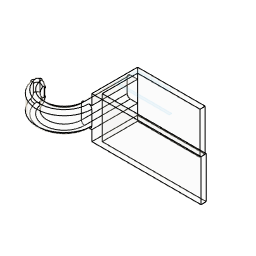
DeskHook v3 (Autodesk Fusion 360 design; units mm, degrees)
Autodesk Fusion 360 part; units mm, degrees
sketch "Sketch1" plane through (0, 0, 0) normal (0, 0, 1) x (1, 0, 0)
  line L0 (5.7833, 3.3448) -> (5.7833, 20.3448)
  line L1 (5.7833, 20.3448) -> (35.7833, 20.3448)
  line L2 (5.7833, 3.3448) -> (55.7833, 3.3448)
  line L3 (35.7833, 20.3448) -> (5.7833, 20.3448)
  line L4 (5.7833, 20.3448) -> (5.7833, 22.8448)
  line L5 (5.7833, 22.8448) -> (35.7833, 22.8448)
  line L6 (35.7833, 22.8448) -> (35.7833, 20.3448)
  line L7 (5.7833, 3.3448) -> (55.7833, 3.3448)
  line L8 (55.7833, 3.3448) -> (55.7833, 0.8448)
  line L9 (55.7833, 0.8448) -> (5.7833, 0.8448)
  line L10 (5.7833, 0.8448) -> (5.7833, 3.3448)
  line L11 (5.7833, 22.8448) -> (3.2833, 22.8448)
  line L12 (3.2833, 22.8448) -> (3.2833, 0.8448)
  line L13 (3.2833, 0.8448) -> (5.7833, 0.8448)
  line L14 (5.7833, 0.8448) -> (5.7833, 22.8448)
  dimension "d1" = 17
  dimension "d2" = 30
  dimension "d3" = 50
  dimension "d4" = 2.5
  dimension "d5" = 2.5
  dimension "d6" = 2.5
  constraint vertical L0
  constraint perpendicular L0 L1
  constraint perpendicular L0 L2
  constraint horizontal L3
  constraint vertical L4
  constraint horizontal L5
  constraint vertical L6
  constraint horizontal L7
  constraint vertical L8
  constraint horizontal L9
  constraint vertical L10
  constraint horizontal L11
  constraint vertical L12
  constraint horizontal L13
  constraint vertical L14
  measures "d1" distance of L0.start L0.end
  measures "d2" distance of L0.end L1.end
  measures "d3" distance of L0.start L2.end
  measures "d4" distance of L1.end L5.end
  measures "d5" distance of L0.start L9.end
  measures "d6" distance of L4.end L11.end
extrude "Extrude1" add sketch "Sketch1" along normal blind 20
sketch "Sketch2" plane through (0, 0, 20) normal (0, 0, 1) x (-1, 0, 0)
  line L0 (-35.7833, -22.8448) -> (-3.2833, -22.8448)
  line L1 (-3.2833, -22.8448) -> (-3.2833, -0.8448)
  line L2 (-3.2833, -0.8448) -> (-55.7833, -0.8448)
  line L3 (-55.7833, -0.8448) -> (-55.7833, -3.3448)
  line L4 (-55.7833, -3.3448) -> (-5.7833, -3.3448)
  line L5 (-5.7833, -3.3448) -> (-5.7833, -20.3448)
  line L6 (-5.7833, -20.3448) -> (-35.7833, -20.3448)
  line L7 (-35.7833, -20.3448) -> (-35.7833, -22.8448)
sketch "Sketch3" plane through (3.2833, 0, 0) normal (-1, 0, 0) x (0, -1, 0)
  line L0 (-22.8448, 0) -> (-0.8448, 0)
  line L1 (-0.8448, 0) -> (-0.8448, 20)
  line L2 (-0.8448, 20) -> (-22.8448, 20)
  line L3 (-22.8448, 20) -> (-22.8448, 0)
  line L4 (-22.8448, 5) -> (-0.8448, 5)
  line L5 (-0.8448, 5) -> (-0.8448, 15)
  line L6 (-0.8448, 15) -> (-22.8448, 15)
  line L7 (-22.8448, 15) -> (-22.8448, 5)
  dimension "d10" = 10
  constraint horizontal L4
  constraint vertical L5
  constraint horizontal L6
  constraint vertical L7
  measures "d10" distance of L4.start L6.end
extrude "Extrude2" add sketch "Sketch3" along normal blind 5 contours L1 L3 L4 L5 L6 L7
sketch "Sketch4" plane through (0, 0, 15) normal (0, 0, 1) x (-1, 0, 0)
  line L0 (-3.2833, -0.8448) -> (-3.2833, -22.8448)
  line L1 (-3.2833, -22.8448) -> (1.7167, -22.8448)
  line L2 (1.7167, -22.8448) -> (1.7167, -0.8448)
  line L3 (1.7167, -0.8448) -> (-3.2833, -0.8448)
  arc A0 (18.2167, -0.8448) -> (1.7167, -0.8448) centre (9.9667, -0.8448) ccw
  line L4 (18.2167, -0.8448) -> (23.2167, -0.8448)
  arc A1 (23.2167, -0.8448) -> (-3.2833, -0.8448) centre (9.9667, -0.8448) ccw
  dimension "d13" = 16.5
  dimension "d14" = 5
  constraint tangent L2 A0
  constraint coincident L2.end L3.start
  constraint horizontal L4
  constraint tangent L0 A1
  constraint coincident L0.start L3.end
  measures "d13" distance of L2.end A0.start
  measures "d14" distance of A0.start L4.end
extrude "Extrude3" add sketch "Sketch4" against normal blind 10 contours L3 A0 L4 A1
fillet "Fillet1" radius 1.5 10 edges at (-20.7167, 0.8448, 15) (-20.7167, 0.8448, 5) (-18.2167, 0.8448, 10) (-23.2167, 0.8448, 10) (-9.9667, -12.4052, 5) (-9.9667, -12.4052, 15) (-9.9667, -7.4052, 5) (-1.7167, 11.8448, 5) (-9.9667, -7.4052, 15) (-1.7167, 11.8448, 15)
scale "Scale1" factor 2 about (5.7833, 20.3448, 20) bodies 1
